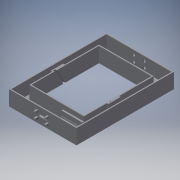
# Autodesk Inventor part: Frame V2.1
Saved by Autodesk Inventor 2018.3 (Build 223284000, 284)
## iProperties
Created: 2020-11-27
Part Number: Frame V2.1
Material: Generic
Document SubType Name: Modeling
Designer: daanv
Density: 1 g/cm^3
Appearance: Default
Author: daanv
## iProperties of the stored document Frame V2_3DPrint.ipt
Created: 2020-12-01
Part Number: Frame V2_3DPrint
Material: Generic
Document SubType Name: Modeling
Designer: daanv
Density: 1 g/cm^3
Appearance: Default
Author: daanv
Autodesk Inventor part; units mm, degrees
ref_plane "YZ Plane" through (0, 0, 0) normal (1, 0, 0) x (0, 1, 0)
ref_plane "XZ Plane" through (0, 0, 0) normal (0, 1, 0) x (-1, 0, 0)
ref_plane "XY Plane" through (0, 0, 0) normal (0, 0, 1) x (1, 0, 0)
sketch "Sketch1" plane through (0, 0, 0) normal (0, 0, 1) x (1, 0, 0)
  line L0 (0, 0) -> (90, 0)
  line L1 (90, 0) -> (90, 130)
  line L2 (90, 130) -> (0, 130)
  line L3 (0, 130) -> (0, 0)
  line L4 (10, 20) -> (80, 20)
  line L5 (80, 20) -> (80, 110)
  line L6 (80, 110) -> (10, 110)
  line L7 (10, 110) -> (10, 20)
  dimension "d0" = 90
  dimension "d1" = 130
  dimension "d2" = 70
  dimension "d3" = 90
  dimension "d16" = 20
  dimension "d17" = 20
  dimension "d18" = 10
  constraints: 16 end point, 4 parallel, 2 horizontal, 2 perpendicular
  measures "d0" distance of L2.end L1.end
  measures "d1" distance of L1.end L0.end
  measures "d2" distance of L6.end L5.end
  measures "d3" distance of L5.end L4.end
  measures "d16" distance between parallel lines of L2 L6
  measures "d17" distance between parallel lines of L0 L4
  measures "d18" distance between parallel lines of L1 L5
extrude "Extrusion1" add sketch "Sketch1" along normal blind 20
sketch "Sketch2" plane through (10, 20, 0) normal (1, 0, 0) x (0, 0, -1)
  line L0 (0, 90) -> (0, 0) projected
  line L1 (0, 42.1132) -> (-20, 30.5662)
  line L2 (-20, 110) -> (-20, -20) projected
  line L3 (0, 42.1132) -> (23.094, 42.1132) construction
  line L4 (-20, 30.5662) -> (-20, 33.5662)
  line L5 (-20, 33.5662) -> (0, 45.1132)
  line L6 (0, 42.1132) -> (0, 45.1132)
  point P0 (-20, 0)
  point P1 (0, -20)
  dimension "d6" = 210
  dimension "d7" = 3
  dimension "d8" = 26.4711
  constraints: 10 end point, 4 point on line, 1 collinear, 1 equal length, 1 horizontal, 1 parallel
  measures "d7" distance of L1.end L4.end
  measures "d8" distance from line of point (-20, 0) L1
extrude "Extrusion2" cut sketch "Sketch2" against normal blind 2
sketch "Sketch3" plane through (80, 20, 0) normal (-1, 0, 0) x (0, 0, 1)
  line L0 (0, 0) -> (0, 90) projected
  line L1 (20, 90) -> (20, 0) projected
  line L2 (0, 42.1132) -> (20, 30.5662)
  line L3 (0, 42.1132) -> (23.094, 42.1132) construction
  line L4 (20, 30.5662) -> (20, 33.5662)
  line L5 (20, 33.5662) -> (0, 45.1132)
  line L6 (0, 42.1132) -> (0, 45.1132)
  point P0 (0, -20)
  dimension "d11" = 30
  dimension "d12" = 3
  dimension "d13" = 26.4711
  constraints: 10 end point, 4 point on line, 1 equal length, 1 horizontal, 1 parallel
  measures "d11" angle of L2 L3
  measures "d12" distance of L2.end L4.end
  measures "d13" distance from line of L1.end L2
extrude "Extrusion3" cut sketch "Sketch3" against normal blind 2
sketch "Sketch4" plane through (0, 0, 0) normal (0, -1, 0) x (1, 0, 0)
  line L0 (0, 0) -> (90, 0) projected
  line L1 (90, 0) -> (90, 20) projected
  line L2 (0, 20) -> (90, 20) projected
  line L3 (0, 0) -> (0, 20) projected
  line L4 (55, 3) -> (35, 3)
  line L5 (35, 3) -> (35, 17)
  line L6 (35, 17) -> (55, 17)
  line L7 (55, 17) -> (55, 3)
  line L8 (53.2053, 7.41) -> (53.87, 5.3643)
  line L9 (53.87, 5.3643) -> (52.1298, 4.1)
  line L10 (52.1298, 4.1) -> (50.3897, 5.3643)
  line L11 (50.3897, 5.3643) -> (51.0543, 7.41)
  line L12 (51.0543, 7.41) -> (53.2053, 7.41)
  line L13 (38.9443, 7.41) -> (39.609, 5.3643)
  line L14 (39.609, 5.3643) -> (37.8689, 4.1)
  line L15 (37.8689, 4.1) -> (36.1287, 5.3643)
  line L16 (36.1287, 5.3643) -> (36.7934, 7.41)
  line L17 (36.7934, 7.41) -> (38.9443, 7.41)
  line L18 (38.9447, 15.55) -> (39.6093, 13.5043)
  line L19 (39.6093, 13.5043) -> (37.8692, 12.24)
  line L20 (37.8692, 12.24) -> (36.129, 13.5043)
  line L21 (36.129, 13.5043) -> (36.7937, 15.55)
  line L22 (36.7937, 15.55) -> (38.9447, 15.55)
  line L23 (53.2053, 15.55) -> (53.87, 13.5043)
  line L24 (53.87, 13.5043) -> (52.1298, 12.24)
  line L25 (52.1298, 12.24) -> (50.3897, 13.5043)
  line L26 (50.3897, 13.5043) -> (51.0543, 15.55)
  line L27 (51.0543, 15.55) -> (53.2053, 15.55)
  point P0 (52.1298, 5.9297)
  point P1 (37.8689, 5.9297)
  point P2 (37.8692, 14.0697)
  point P3 (52.1298, 14.0697)
  dimension "d19" = 20
  dimension "d20" = 14
  dimension "d21" = 3
  dimension "d22" = 3
  dimension "d23" = 35
  dimension "d24" = 35
  dimension "d25" = 1.45
  dimension "d26" = 1.45
  dimension "d27" = 1.1
  dimension "d28" = 1.1
  dimension "d29" = 12.11
  dimension "d30" = 1.13
  dimension "d31" = 1.13
  dimension "d32" = 4.83
  dimension "d33" = 4.83
  dimension "d34" = 1.129
  dimension "d35" = 1.1287
  constraints: 48 end point, 5 horizontal, 3 equal length, 2 parallel, 1 perpendicular, 44 other
  measures "d19" distance of L5.end L6.end
  measures "d20" distance of L4.end L5.end
  measures "d21" distance between parallel lines of L4 L0
  measures "d22" distance between parallel lines of L2 L6
  measures "d23" distance between parallel lines of L1 L7
  measures "d24" distance between parallel lines of L3 L5
  measures "d25" distance between parallel lines of L6 L27
  measures "d26" distance between parallel lines of L22 L6
  measures "d27" distance from line of L4 L9.end
  measures "d28" distance from line of L4 L14.end
  measures "d29" distance of L13.start L11.end
  measures "d30" distance from line of L7 L8.end
  measures "d31" distance from line of L7 L23.end
  measures "d32" distance from line of L12 L24.end
  measures "d33" distance from line of L17 L19.end
  measures "d34" distance from line of L5 L20.end
  measures "d35" distance from line of L5 L15.end
extrude "Extrusion4" add sketch "Sketch4" along normal blind 4 contours L8 L9 L10 L11 L12 | L13 L14 L15 L16 L17 | L18 L19 L20 L21 L22 | L23 L24 L25 L26 L27
chamfer "Chamfer1" distance 0.5 angle 45 20 edges at (52.1298, -4, 15.55) (50.722, -4, 14.5272) (51.2597, -4, 12.8722) (52.9999, -4, 12.8722) (53.5377, -4, 14.5272) (52.1298, -4, 7.41) (53.5377, -4, 6.3872) (52.9999, -4, 4.7322) (51.2597, -4, 4.7322) (50.722, -4, 6.3872) (39.277, -4, 14.5272) (38.7393, -4, 12.8722) (36.9991, -4, 12.8722) (36.4613, -4, 14.5272) (37.8692, -4, 15.55) (37.8689, -4, 7.41) (39.2767, -4, 6.3872) (38.7389, -4, 4.7322) (36.9988, -4, 4.7322) (36.461, -4, 6.3872)
sketch "Sketch5" plane through (0, 130, 0) normal (0, 1, 0) x (1, 0, 0)
  line L0 (90, 0) -> (0, 0) projected
  line L1 (0, 0) -> (0, -20) projected
  line L2 (90, -20) -> (0, -20) projected
  line L3 (90, 0) -> (90, -20) projected
  line L4 (55, -17) -> (35, -17)
  line L5 (35, -17) -> (35, -3)
  line L6 (35, -3) -> (55, -3)
  line L7 (55, -3) -> (55, -17)
  line L8 (52.1306, -7.7585) -> (50.3912, -6.4948)
  line L9 (50.3912, -6.4948) -> (51.0556, -4.45)
  line L10 (51.0556, -4.45) -> (53.2056, -4.45)
  line L11 (53.2056, -4.45) -> (53.87, -6.4948)
  line L12 (53.87, -6.4948) -> (52.1306, -7.7585)
  line L13 (52.1306, -15.9) -> (50.3912, -14.6363)
  line L14 (50.3912, -14.6363) -> (51.0556, -12.5915)
  line L15 (51.0556, -12.5915) -> (53.2056, -12.5915)
  line L16 (53.2056, -12.5915) -> (53.87, -14.6363)
  line L17 (53.87, -14.6363) -> (52.1306, -15.9)
  line L18 (37.8674, -15.9) -> (36.128, -14.6363)
  line L19 (36.128, -14.6363) -> (36.7924, -12.5915)
  line L20 (36.7924, -12.5915) -> (38.9424, -12.5915)
  line L21 (38.9424, -12.5915) -> (39.6068, -14.6363)
  line L22 (39.6068, -14.6363) -> (37.8674, -15.9)
  line L23 (37.8674, -7.7585) -> (36.128, -6.4948)
  line L24 (36.128, -6.4948) -> (36.7924, -4.45)
  line L25 (36.7924, -4.45) -> (38.9424, -4.45)
  line L26 (38.9424, -4.45) -> (39.6068, -6.4948)
  line L27 (39.6068, -6.4948) -> (37.8674, -7.7585)
  point P0 (52.1306, -5.9296)
  point P1 (52.1306, -14.0711)
  point P2 (37.8674, -14.0711)
  point P3 (37.8674, -5.9296)
  dimension "d41" = 20
  dimension "d42" = 14
  dimension "d43" = 3
  dimension "d44" = 3
  dimension "d45" = 35
  dimension "d46" = 35
  dimension "d141" = 1.45
  dimension "d142" = 2.15
  dimension "d143" = 1.13
  dimension "d144" = 2.15
  dimension "d145" = 1.13
  dimension "d146" = 1.1
  dimension "d148" = 2.15
  dimension "d149" = 1.1
  dimension "d150" = 1.128
  dimension "d151" = 4.833
  dimension "d153" = 12.1132
  dimension "d154" = 2.15
  dimension "d155" = 1.128
  dimension "d156" = 1.45
  dimension "d157" = 4.833
  dimension "d158" = 12.1132
  constraints: 48 end point, 4 horizontal, 2 parallel, 1 perpendicular, 44 other
  measures "d41" distance of L5.end L6.end
  measures "d42" distance of L4.end L5.end
  measures "d43" distance between parallel lines of L2 L4
  measures "d44" distance between parallel lines of L0 L6
  measures "d45" distance between parallel lines of L3 L7
  measures "d46" distance between parallel lines of L1 L5
  measures "d141" distance between parallel lines of L6 L10
  measures "d142" distance of L9.end L10.end
  measures "d143" distance from line of L7 L11.end
  measures "d144" distance of L14.end L15.end
  measures "d145" distance from line of L7 L16.end
  measures "d146" distance from line of L4 L13.start
  measures "d148" distance of L19.end L20.end
  measures "d149" distance from line of L4 L18.start
  measures "d150" distance from line of L5 L18.end
  measures "d151" distance from line of L8.start L15
  measures "d153" distance of L20.end L14.end
  measures "d154" distance of L24.end L25.end
  measures "d155" distance from line of L5 L23.end
  measures "d156" distance between parallel lines of L6 L25
  measures "d157" distance from line of L23.start L20
  measures "d158" distance of L25.end L9.end
extrude "Extrusion5" cut sketch "Sketch5" against normal blind 4 contours L8 L9 L10 L11 L12 | L13 L14 L15 L16 L17 | L18 L19 L20 L21 L22 | L23 L24 L25 L26 L27
chamfer "Chamfer2" distance 0.5 angle 45 20 edges at (51.2609, 130, 15.2681) (53.0003, 130, 15.2681) (53.5378, 130, 13.6139) (52.1306, 130, 12.5915) (50.7234, 130, 13.6139) (51.2609, 130, 7.1266) (53.0003, 130, 7.1266) (53.5378, 130, 5.4724) (52.1306, 130, 4.45) (50.7234, 130, 5.4724) (39.2746, 130, 13.6139) (38.7371, 130, 15.2681) (36.9977, 130, 15.2681) (36.4602, 130, 13.6139) (37.8674, 130, 12.5915) (36.9977, 130, 7.1266) (38.7371, 130, 7.1266) (39.2746, 130, 5.4724) (37.8674, 130, 4.45) (36.4602, 130, 5.4724)
sketch "Sketch6" plane through (0, 0, 20) normal (0, 0, 1) x (1, 0, 0)
  line L0 (0, 0) -> (90, 0) projected
  line L1 (90, 0) -> (90, 130) projected
  line L2 (90, 130) -> (0, 130) projected
  line L3 (1.5, 130) -> (1.5, 1.5)
  line L4 (0, 0) -> (90, 0) projected
  line L5 (1.5, 1.5) -> (88.5, 1.5)
  line L6 (88.5, 1.5) -> (88.5, 128.5)
  line L7 (88.5, 128.5) -> (1.5, 128.5)
  line L8 (8.5, 111.5) -> (8.5, 65.5)
  line L9 (10, 65.1132) -> (8, 65.1132) projected
  line L10 (8.5, 65.5) -> (6.5, 65.5)
  line L11 (6.5, 65.5) -> (6.5, 49.066)
  line L12 (6.5, 49.066) -> (8.5, 49.066)
  line L13 (8.5, 49.066) -> (8.5, 18.5)
  line L14 (8.5, 18.5) -> (81.5, 18.5)
  line L15 (81.5, 18.5) -> (81.5, 49.066)
  line L16 (81.5, 49.066) -> (83.5, 49.066)
  line L17 (83.5, 49.066) -> (83.5, 65.5)
  line L18 (83.5, 65.5) -> (81.5, 65.5)
  line L19 (81.5, 65.5) -> (81.5, 111.5)
  line L20 (81.5, 111.5) -> (8.5, 111.5)
  dimension "d79" = 128.5
  dimension "d80" = 87
  dimension "d81" = 127
  dimension "d82" = 46
  dimension "d83" = 2
  dimension "d84" = 16.434
  dimension "d85" = 2
  dimension "d86" = 30.566
  dimension "d87" = 73
  dimension "d88" = 2
  constraints: 32 end point, 10 perpendicular, 6 point on line, 2 parallel, 1 horizontal
  measures "d79" distance of L3.start L3.end
  measures "d80" distance of L3.end L5.end
  measures "d81" distance of L5.end L6.end
  measures "d82" distance of L8.start L8.end
  measures "d83" distance of L8.end L10.end
  measures "d84" distance of L10.end L11.end
  measures "d85" distance of L11.end L12.end
  measures "d86" distance of L12.end L13.end
  measures "d87" distance of L13.end L14.end
  measures "d88" distance of L15.end L16.end
extrude "Extrusion6" cut sketch "Sketch6" against normal blind 18
sketch "Sketch7" plane through (0, 0, 0) normal (0, -1, 0) x (1, 0, 0)
  line L0 (0, 0) -> (90, 0) projected
  line L1 (90, 0) -> (90, 20) projected
  line L2 (0, 20) -> (90, 20) projected
  line L3 (0, 0) -> (0, 20) projected
  line L4 (39.5, 8.7) -> (50.5, 8.7)
  line L5 (50.5, 8.7) -> (50.5, 11.3)
  line L6 (50.5, 11.3) -> (39.5, 11.3)
  line L7 (39.5, 11.3) -> (39.5, 8.7)
  dimension "d100" = 11
  dimension "d101" = 2.6
  dimension "d102" = 8.7
  dimension "d103" = 39.5
  dimension "d104" = 39.5
  dimension "d105" = 8.7
  constraints: 8 end point, 2 parallel, 1 horizontal, 1 perpendicular
  measures "d100" distance of L4.start L4.end
  measures "d101" distance of L4.end L5.end
  measures "d102" distance between parallel lines of L2 L6
  measures "d103" distance between parallel lines of L3 L7
  measures "d104" distance between parallel lines of L1 L5
  measures "d105" distance between parallel lines of L0 L4
extrude "Extrusion7" cut sketch "Sketch7" against normal blind 10 contours L7 L6 L5 L4
sketch "Sketch8" plane through (8.5, 18.5, 20) normal (0, -1, 0) x (1, 0, 0)
  line L0 (0, 0) -> (73, 0) projected
  line L1 (0, -18) -> (73, -18) projected
  line L2 (73, 0) -> (73, -18) projected
  line L3 (73, -6) -> (45, -6)
  line L4 (45, -6) -> (45, -18)
  line L5 (45, -18) -> (73, -18)
  line L6 (73, -18) -> (73, -6)
  point P0 (-8.5, -20)
  dimension "d108" = 28
  dimension "d109" = 6
  constraints: 8 end point, 2 parallel, 2 point on line, 1 horizontal, 1 perpendicular
  measures "d108" distance of L5.end L4.end
  measures "d109" distance between parallel lines of L0 L3
extrude "Extrusion8" add sketch "Sketch8" along normal blind 2.2
sketch "Sketch9" plane through (1.5, 1.5, 20) normal (0, 1, 0) x (1, 0, 0)
  line L0 (87, 0) -> (87, 18) projected
  line L1 (87, 18) -> (0, 18) projected
  line L2 (80, 18) -> (52, 18)
  line L3 (52, 18) -> (52, 6)
  line L4 (52, 6) -> (80, 6)
  line L5 (80, 6) -> (80, 18)
  point P0 (-1.5, 20)
  dimension "d114" = 28
  dimension "d115" = 12
  dimension "d116" = 7
  constraints: 8 end point, 2 parallel, 1 horizontal, 1 perpendicular, 1 point on line
  measures "d114" distance of L4.end L3.end
  measures "d115" distance of L3.end L2.end
  measures "d116" distance between parallel lines of L0 L5
extrude "Extrusion9" add sketch "Sketch9" along normal blind 2.2
sketch "Sketch10" plane through (1.5, 3.7, 20) normal (0, 1, 0) x (1, 0, 0)
  line L0 (80, 6) -> (80, 18) projected
  line L1 (52, 18) -> (52, 6) projected
  line L2 (52, 6) -> (80, 6) projected
  line L3 (52, 15.8) -> (80, 15.8)
  line L4 (80, 15.8) -> (80, 14.8)
  line L5 (80, 14.8) -> (52, 14.8)
  line L6 (52, 14.8) -> (52, 15.8)
  line L7 (80, 13) -> (52, 13)
  line L8 (52, 13) -> (52, 12)
  line L9 (52, 12) -> (80, 12)
  line L10 (80, 12) -> (80, 13)
  point P0 (-1.5, 20)
  dimension "d119" = 1
  dimension "d120" = 0
  dimension "d121" = 8.8
  dimension "d122" = 1
  dimension "d123" = 6
  constraints: 16 end point, 4 parallel, 2 horizontal, 2 perpendicular, 2 point on line, 1 midpoint
  measures "d119" distance of L3.end L4.end
  measures "d120" distance between parallel lines of L0 L4
  measures "d121" distance between parallel lines of L2 L5
  measures "d122" distance of L8.end L7.end
  measures "d123" distance between parallel lines of L2 L9
extrude "Extrusion10" add sketch "Sketch10" along normal blind 0.55 contours L9 L1 L7 L0 | L5 L1 L3 L0
sketch "Sketch11" plane through (1.5, 3.7, 20) normal (0, 1, 0) x (1, 0, 0)
  line L0 (52, 13) -> (80, 13) projected
  line L1 (80, 13) -> (80, 14.8) projected
  line L2 (80, 14.8) -> (52, 14.8) projected
  line L3 (52, 14.8) -> (52, 13) projected
  point P0 (-1.5, 20)
extrude "Extrusion11" cut sketch "Sketch11" against normal blind 0.6
sketch "Sketch12" plane through (8.5, 16.3, 20) normal (0, -1, 0) x (1, 0, 0)
  line L0 (73, -6) -> (45, -6) projected
  line L1 (45, -6) -> (45, -18) projected
  line L2 (73, -18) -> (73, -6) projected
  line L3 (45, -16) -> (73, -16)
  line L4 (73, -16) -> (73, -15)
  line L5 (73, -15) -> (45, -15)
  line L6 (45, -15) -> (45, -16)
  line L7 (45, -13.2) -> (73, -13.2)
  line L8 (73, -13.2) -> (73, -12.2)
  line L9 (73, -12.2) -> (45, -12.2)
  line L10 (45, -12.2) -> (45, -13.2)
  point P0 (-8.5, -20)
  dimension "d128" = 1
  dimension "d129" = 1
  dimension "d130" = 6.2
  dimension "d131" = 1.8
  constraints: 16 end point, 4 parallel, 4 point on line, 2 horizontal, 2 perpendicular
  measures "d128" distance of L4.end L3.end
  measures "d129" distance of L8.end L7.end
  measures "d130" distance between parallel lines of L0 L9
  measures "d131" distance between parallel lines of L7 L5
extrude "Extrusion12" add sketch "Sketch12" along normal blind 0.55 contours L2 L7 L1 L9 | L2 L3 L1 L5
sketch "Sketch13" plane through (8.5, 16.3, 20) normal (0, -1, 0) x (1, 0, 0)
  line L0 (45, -15) -> (73, -15) projected
  line L1 (73, -15) -> (73, -13.2) projected
  line L2 (73, -13.2) -> (45, -13.2) projected
  line L3 (45, -13.2) -> (45, -15) projected
  point P0 (-8.5, -20)
extrude "Extrusion13" cut sketch "Sketch13" against normal blind 0.6
sketch "Sketch14" plane through (81.5, 1.5, 14) normal (1, 0, 0) x (0, 0, -1)
  line L0 (8.8, 2.75) -> (8.8, 1.6) projected
  line L1 (8.8, 1.6) -> (7, 1.6) projected
  line L2 (7, 1.6) -> (7, 2.75) projected
  line L3 (6, 2.75) -> (7, 2.75) projected
  line L4 (6, 2.2) -> (6, 2.75) projected
  line L5 (0, 2.2) -> (6, 2.2) projected
  line L6 (0, 0) -> (0, 2.2) projected
  line L7 (12, 0) -> (0, 0) projected
  line L8 (12, 2.2) -> (12, 0) projected
  line L9 (9.8, 2.2) -> (12, 2.2) projected
  line L10 (9.8, 2.2) -> (9.8, 2.75) projected
  line L11 (8.8, 2.75) -> (9.8, 2.75) projected
  point P0 (14, -1.5)
extrude "Extrusion14" add sketch "Sketch14" along normal blind 7
chamfer "Chamfer3" distance 6 angle 10 1 edges at (88.5, 3.1, 6.1) measured on face at (76.8333, 3.1, 5.8)
body "Solid1"
